Autodesk Inventor part; units mm, degrees
(part 2 of 2)
sketch "Náčrt65" plane through (0, 0, 0) normal (0, -1, 0) x (1, 0, 0)
  line L0 (24, -49.75) -> (-24, -49.75) projected
  line L1 (3, -48.75) -> (-12, -48.75)
  line L2 (-12, -48.75) -> (-12, -40)
  line L3 (-12, -40) -> (3, -40)
  line L4 (3, -40) -> (3, -49.75)
  circle A0 centre (-0.7, -44.375) radius 1.65
  line L5 (-0.7, -44.375) -> (-12, -48.75) construction
  line L6 (-0.7, -44.375) -> (-12, -40) construction
  line L7 (24, -36.6665) -> (6, -36.6665) projected
  line L8 (24, -39.3886) -> (24, -36.6665) projected
  line L9 (-24, -39.3886) -> (24, -39.3886) projected
  line L10 (-24, -39.3886) -> (-24, -36.6665) projected
  line L11 (-24, -36.6665) -> (-6, -36.6665) projected
  line L12 (6, -36.6665) -> (-6, -36.6665) projected
  line L13 (-6, -36.6665) -> (6, -36.6665) projected
  line L14 (-6, -36.6665) -> (-6, -29.8335) projected
  line L15 (-6, -29.8335) -> (-14, -29.8335) projected
  line L16 (-14, -29.8335) -> (-14, -14) projected
  line L17 (14, -14) -> (-14, -14) projected
  line L18 (14, -29.8335) -> (14, -14) projected
  line L19 (6, -29.8335) -> (14, -29.8335) projected
  line L20 (6, -36.6665) -> (6, -29.8335) projected
  line L21 (24, -36.6665) -> (6, -36.6665) projected
  line L22 (6, -36.6665) -> (6, -29.8335) projected
  line L23 (14, -29.8335) -> (6, -29.8335) projected
  line L24 (24, -29.8335) -> (14, -29.8335) projected
  line L25 (24, -36.6665) -> (24, -29.8335) projected
  line L26 (-24, -36.6665) -> (-6, -36.6665) projected
  line L27 (-24, -36.6665) -> (-24, -29.8335) projected
  line L28 (-24, -29.8335) -> (-14, -29.8335) projected
  line L29 (-14, -29.8335) -> (-6, -29.8335) projected
  line L30 (-6, -36.6665) -> (-6, -29.8335) projected
  circle A1 centre (8, -43.2692) radius 3.75 projected
  circle A2 centre (-19, -43.5625) radius 1.75 projected
  circle A3 centre (19, -43.5625) radius 1.75 projected
  line L31 (-24, -39.3886) -> (24, -39.3886) projected
  line L32 (24, -39.3886) -> (24, -49.75) projected
  line L33 (24, -49.75) -> (-24, -49.75) projected
  line L34 (-24, -39.3886) -> (-24, -49.75) projected
  line L35 (3, -40) -> (3, -36.6665)
  line L36 (-4.4, -36.6665) -> (-4.4, -44.375)
  line L37 (-4.4, -44.375) -> (-0.7, -44.375) construction
  line L38 (-0.7, -44.375) -> (3, -44.375) construction
  line L39 (-4, -49.75) -> (-4, -48.75)
  line L40 (-12, -48.75) -> (-12, -49.75)
  line L41 (3, -43.5) -> (-12, -43.5)
  circle A4 centre (-0.7, -44.375) radius 4
  line L42 (3, -48.95) -> (-4, -48.95)
  circle A5 centre (-0.7, -29.375) radius 1.65
  line L43 (-0.7, -29.375) -> (-0.7, -44.375) construction
  line L44 (-5.2, -29.375) -> (-5.2, -44.375)
  line L45 (3.8, -44.375) -> (3.8, -29.375)
  arc A6 (3.8, -29.375) -> (-5.2, -29.375) centre (-0.7, -29.375) ccw
  arc A7 (-5.2, -44.375) -> (3.8, -44.375) centre (-0.7, -44.375) ccw
  line L46 (3.2031, -43.5) -> (3, -42.5939)
  circle A8 centre (-0.7, -29.375) radius 4.5
  circle A9 centre (-0.7, -44.375) radius 5
  line L47 (3, -47.75) -> (-4, -47.75)
  line L48 (-4, -47.75) -> (-4, -48.75)
  line L49 (-3, -41.1024) -> (-3, -39.3886)
  point P0 (0, 0)
  point P1 (-10.75, -49.75)
  point P2 (-4.4, -40)
  point P3 (-4.6031, -43.5)
  point P4 (2.6889, -43.5)
  point P5 (-0.7, -36.875)
  point P6 (-5.2, -36.6665)
  point P7 (3.8, -36.6665)
  point P8 (-5.2, -40)
  point P9 (3, -46.9362)
  point P10 (-5.2, -39.3886)
  point P11 (3.8, -39.3886)
  point P12 (-2.7173, -48.95)
  point P13 (1.3173, -48.95)
  point P14 (3, -47.738)
  point P15 (3.8, -42.1956)
  point P16 (1.7206, -48.75)
  point P17 (-3.1206, -48.75)
  point P18 (2.2765, -47.75)
  point P19 (1.4469, -47.75)
  point P20 (-4.4, -43.5)
  point P21 (-3, -40)
  point P22 (3, -42.8551)
  point P23 (3, -45.8949)
  point P24 (-3.6765, -47.75)
  point P25 (-2.8469, -47.75)
  point P26 (2.9891, -47.75)
  dimension "d309" = 15
  dimension "d310" = 3
  dimension "d311" = 8.75
  dimension "d312" = 3.3
  dimension "d324" = 1
  dimension "d338" = 3.7
  dimension "d339" = 8
  dimension "d340" = 3.5
  dimension "d341" = 8
  dimension "d344" = 0.8
  dimension "d345" = 3.3
  dimension "d346" = 15
  dimension "d350" = 4.5
  dimension "d384" = 10
  dimension "d385" = 1
  dimension "d386" = 6
  constraints: 44 end point, 16 point on line, 10 perpendicular, 7 centre point, 6 point on circle, 5 tangent, 4 parallel, 3 coincident, 2 equal length, 1 concentric, 1 horizontal, 1 midpoint, 1 vertical, 1 vertical alignment
  measures "d309" distance of L2.end L3.end
  measures "d310" distance from line of point (0, 0) L4
  measures "d311" distance of L1.end L2.end
  measures "d312" diameter of A0
  measures "d324" distance between parallel lines of L0 L1
  measures "d338" distance from line of L4 L5.start
  measures "d339" distance between parallel lines of L40 L39
  measures "d340" distance between parallel lines of L3 L41
  measures "d341" diameter of A4
  measures "d344" distance between parallel lines of L0 L42
  measures "d345" diameter of A5
  measures "d346" distance of L43.start L5.start
  measures "d350" radius of A6
  measures "d384" diameter of A9
  measures "d385" distance between parallel lines of L1 L47
  measures "d386" distance between parallel lines of L49 L4
extrude "Vysunutí70" cut sketch "Náčrt65" against normal through all contours L0 L40 L1 L39 | L42 A9 L1 L4 | L45 A9 L4 L35 L9 | L9 L35 L12 L45 | L39 L1 A9 L42 | L1 A9 L47 L4 | A9 L42 | L42 A9 L1 A7 | L35 L3 A9 L9 | L9 A9 L36 L12 L35 | A9 L4 A7 L45 | L45 A7 L4 A4 L46 A9 | L12 L44 A8 L45 | L2 L41 A9 L48 L1 | L48 A9 L1 | L1 A7 L47 A9 | L47 A9 L4 | A9 L3 L49 L9 | L9 A9 | L4 A9 L3 | L4 A4 L49 L3 A9 | A8 A6 | L2 L3 L44 A9 L41 | A9 L48 L47 A7 L1 | A9 L41 L44 A7 L47 L48 | A7 L1 | L1 A7 L47 A4 | L47 A7 L4 A9 | A9 L49 L9 | L36 L9 L44 L12 | A7 L47 A4 L4 | L46 A4 L4 | L9 L36 L3 L44 | A9 L44 L41 | L49 A9 L3 L36 L9 | L49 L3 A9 | L49 A4 L36 A9 L3 | A4 L47 L41 A0 L4 | L4 A4 | L4 L41 A0 L36 A4 | L3 L36 A9 L44 | L44 A9 L36 A4 L41 | L41 A4 L47 A7 L44 | A4 L47 | A9 L36 L3 | A4 L36 L41 | L41 A0 | A0 L41 | A5
extrude "Vysunutí77" add sketch "Náčrt65" against normal blind 1.5 contours L42 A9 L1 L4 | L45 A9 L4 L35 L9 | L9 L35 L12 L45 | L39 L1 A9 L42 | L1 A9 L47 L4 | A9 L42 | L42 A9 L1 A7 | L35 L3 A9 L9 | L9 A9 L36 L12 L35 | A9 L4 A7 L45 | L45 A7 L4 A4 L46 A9 | L12 L44 A8 L45 | L48 A9 L1 | L1 A7 L47 A9 | L47 A9 L4 | A9 L3 L49 L9 | L9 A9 | L4 A9 L3 | L4 A4 L49 L3 A9 | A8 A6 | A9 L48 L47 A7 L1 | A7 L1 | L1 A7 L47 A4 | L47 A7 L4 A9 | A9 L49 L9 | L36 L9 L44 L12 | A7 L47 A4 L4 | L46 A4 L4 | L9 L36 L3 L44 | L49 A9 L3 L36 L9 | L49 L3 A9 | A5
extrude "Vysunutí79" add sketch "Náčrt65" against normal blind 3 contours L9 L35 L12 L45 | L9 A9 L36 L12 L35 | L12 L44 A8 L45 | L9 A9 | A8 A6 | L36 L9 L44 L12
sketch "Náčrt70" plane through (0, 2, 0) normal (0, 1, 0) x (1, 0, 0)
  line L0 (3.8, 36.6665) -> (3.8, 29.375) projected
  line L1 (-5.2, 29.375) -> (-5.2, 36.6665) projected
  line L2 (-6, 36.6665) -> (-5.2, 36.6665) projected
  line L3 (-6, 36.6665) -> (-6, 29.8335) projected
  line L4 (-6, 29.8335) -> (-14, 29.8335) projected
  line L5 (-14, 29.8335) -> (-14, 14) projected
  line L6 (14, 14) -> (-14, 14) projected
  line L7 (14, 29.8335) -> (14, 14) projected
  line L8 (6, 29.8335) -> (14, 29.8335) projected
  line L9 (6, 36.6665) -> (6, 29.8335) projected
  line L10 (3.8, 36.6665) -> (6, 36.6665) projected
  line L11 (6, 29.8335) -> (3.8, 29.8335)
  line L12 (-6, 29.8335) -> (-5.2, 29.8335)
  arc A0 (-5.2, 29.375) -> (3.8, 29.375) centre (-0.7, 29.375) ccw projected
  point P0 (0, 0)
  constraints: 4 end point, 3 point on line, 1 perpendicular
extrude "Vysunutí81" add sketch "Náčrt70" along normal up to surface (1.9 mm away) contours L10 L9 L11 L0 | L12 L3 L2 L1
sketch "Náčrt72" plane through (0, 0, 0) normal (0, -1, 0) x (1, 0, 0)
  line L0 (6.3401, -40.3942) -> (9.6599, -40.3942) projected
  line L1 (2.125, -32.2) -> (-3.525, -32.2)
  line L2 (-3.525, -32.2) -> (-3.525, -26.55)
  line L3 (-3.525, -26.55) -> (2.125, -26.55)
  line L4 (2.125, -26.55) -> (2.125, -32.2)
  line L5 (2.125, -32.2) -> (-3.525, -26.55) construction
  line L6 (-3.525, -32.2) -> (2.125, -26.55) construction
  arc A0 (3.8, -29.375) -> (-5.2, -29.375) centre (-0.7, -29.375) ccw projected
  point P0 (0, 0)
  dimension "d387" = 5.65
  constraints: 12 end point, 2 midpoint, 2 parallel, 2 perpendicular, 1 horizontal
  measures "d387" distance of L1.end L2.end
extrude "Vysunutí83" cut sketch "Náčrt72" against normal blind 2
chamfer "Zkosení6" distance 0.7 angle 45 1 edges at (-2.35, 2, -29.375)
sketch "Náčrt75" plane through (0, 9, 0) normal (0, 1, 0) x (1, 0, 0)
  line L0 (3.8, 42.1956) -> (3.8, 39.3886) projected
  line L1 (3.8, 39.3886) -> (24, 39.3886) projected
  line L2 (24, 39.3886) -> (24, 49.75) projected
  line L3 (24, 49.75) -> (-4, 49.75) projected
  line L4 (-4, 49.75) -> (-4, 48.95) projected
  line L5 (-4, 48.95) -> (-2.7173, 48.95) projected
  arc A0 (1.3173, 48.95) -> (-2.7173, 48.95) centre (-0.7, 44.375) ccw projected
  line L6 (1.3173, 48.95) -> (3, 48.95) projected
  line L7 (3, 48.95) -> (3, 47.738) projected
  arc A1 (3.8, 42.1956) -> (3, 47.738) centre (-0.7, 44.375) ccw projected
  circle A2 centre (8, 43.2692) radius 3.75 projected
  circle A3 centre (19, 43.5625) radius 1.75 projected
  line L8 (-1.1994, 49.35) -> (-0.2006, 49.35)
  point P0 (0, 0)
  dimension "d397" = 0.4
  constraints: 2 end point, 2 point on circle, 1 horizontal
  measures "d397" distance between parallel lines of L3 L8
extrude "Vysunutí86" add sketch "Náčrt75" against normal up to next contours L8 A0
sketch "Náčrt76" plane through (-5.2, 3.9, -29.8335) normal (1, 0, 0) x (0, 0, -1)
  line L0 (0, -0.9) -> (9.5551, -0.9) projected
  line L1 (9.5551, -0.9) -> (9.5551, -2.4) projected
  line L2 (9.5551, -2.4) -> (10.1665, -2.4) projected
  line L3 (10.1665, -2.4) -> (10.1665, 5.1) projected
  line L4 (9.5551, 5.1) -> (10.1665, 5.1) projected
  arc A0 (6.833, 0) -> (9.5551, 5.1) centre (3.4165, 5.1) ccw projected
  line L5 (0, 0) -> (6.833, 0) projected
  line L6 (0, -0.9) -> (0, 0) projected
  line L7 (6.833, 0) -> (10.1665, 0)
  point P0 (-29.8335, -3.9)
  constraints: 2 end point, 1 perpendicular, 1 point on line
extrude "Vysunutí87" cut sketch "Náčrt76" against normal up to surface (6.8 mm away) contours A0 L4 L3 L7
fillet "Zaoblení2" radius 2 1 edges at (-8.6, 3.9, -40)
fillet "Zaoblení3" radius 0.25 4 edges at (-3, 0.75, -41.1024) (-4, 0.75, -47.75) (-2.8469, 0.75, -47.75) (-3, 0.75, -40)
